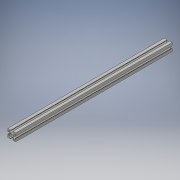
# Autodesk Inventor part: 20 in 80-20 extrusion
Saved by Autodesk Inventor 2016 SP2 (Build 200236200, 236)
## iProperties
Created: 2018-01-11
Part Number: 20 in 80-20 extrusion
Material: Generic
Document SubType Name: Modeling
Designer: CAD
Density: 1 g/cm^3
Appearance: Default
Author: CAD
Autodesk Inventor part; units mm, degrees
ref_plane "YZ Plane" through (0, 0, 0) normal (1, 0, 0) x (0, 1, 0)
ref_plane "XZ Plane" through (0, 0, 0) normal (0, 1, 0) x (-1, 0, 0)
ref_plane "XY Plane" through (0, 0, 0) normal (0, 0, 1) x (1, 0, 0)
sketch "Sketch1" plane through (0, 0, 0) normal (0, 0, 1) x (1, 0, 0)
  line L0 (-12.7, 12.7) -> (12.7, 12.7)
  line L1 (12.7, 12.7) -> (12.7, -12.7)
  line L2 (12.7, -12.7) -> (-12.7, -12.7)
  line L3 (-12.7, -12.7) -> (-12.7, 12.7)
  point P0 (0, 0)
  dimension "d0" = 25.4
  dimension "d1" = 25.4
  dimension "d2" = 12.7
  dimension "d3" = 12.7
  constraints: 8 end point, 2 parallel, 1 horizontal, 1 perpendicular
  measures "d0" distance of L1.end L2.end
  measures "d1" distance of L0.end L1.end
  measures "d2" distance from line of L1 point (0, 0)
  measures "d3" distance from line of point (0, 0) L0
extrude "Extrusion1" add sketch "Sketch1" along normal blind 508
sketch "Sketch2" plane through (0, 0, 508) normal (0, 0, 1) x (1, 0, 0)
  circle A0 centre (0, 0) radius 2.54
  line L0 (-4.5085, 4.5085) -> (4.5085, 4.5085)
  line L1 (-4.5085, -4.5085) -> (4.5085, -4.5085)
  line L2 (4.5085, 4.5085) -> (4.5085, -4.5085)
  line L3 (-4.5085, 4.5085) -> (-4.5085, -4.5085)
  line L4 (-3.0896, 4.5085) -> (-11.2811, 12.7)
  line L5 (-4.5085, 3.0537) -> (-12.7, 11.2452)
  line L6 (12.7, 12.7) -> (-12.7, 12.7) projected
  line L7 (-12.7, 12.7) -> (-12.7, 4.0005)
  line L8 (-10.668, 4.0005) -> (-10.668, 9.2132)
  line L9 (-9.2491, 10.668) -> (-3.3655, 10.668)
  line L10 (-12.7, 12.7) -> (-3.3655, 12.7)
  line L11 (-2.7305, 11.303) -> (-2.7305, 12.065)
  line L12 (-12.065, 3.3655) -> (-11.303, 3.3655)
  arc A1 (-12.7, 4.0005) -> (-12.065, 3.3655) centre (-12.065, 4.0005) ccw
  arc A2 (-11.303, 3.3655) -> (-10.668, 4.0005) centre (-11.303, 4.0005) ccw
  arc A3 (-3.3655, 10.668) -> (-2.7305, 11.303) centre (-3.3655, 11.303) ccw
  arc A4 (-2.7305, 12.065) -> (-3.3655, 12.7) centre (-3.3655, 12.065) ccw
  arc A5 (-3.3655, -11.303) -> (-4.0005, -10.668) centre (-4.0005, -11.303) ccw
  line L13 (-3.3655, -12.065) -> (-3.3655, -11.303)
  arc A6 (-4.0005, -12.7) -> (-3.3655, -12.065) centre (-4.0005, -12.065) ccw
  line L14 (-3.0537, -4.5085) -> (-11.2452, -12.7)
  line L15 (-10.668, -9.2491) -> (-10.668, -3.3655)
  line L16 (-4.5085, -3.0896) -> (-12.7, -11.2811)
  line L17 (-12.7, -12.7) -> (-12.7, -3.3655)
  arc A7 (-10.668, -3.3655) -> (-11.303, -2.7305) centre (-11.303, -3.3655) ccw
  line L18 (-11.303, -2.7305) -> (-12.065, -2.7305)
  arc A8 (-12.065, -2.7305) -> (-12.7, -3.3655) centre (-12.065, -3.3655) ccw
  line L19 (-4.0005, -10.668) -> (-9.2132, -10.668)
  line L20 (-12.7, -12.7) -> (-4.0005, -12.7)
  arc A9 (11.303, -3.3655) -> (10.668, -4.0005) centre (11.303, -4.0005) ccw
  line L21 (12.065, -3.3655) -> (11.303, -3.3655)
  arc A10 (12.7, -4.0005) -> (12.065, -3.3655) centre (12.065, -4.0005) ccw
  line L22 (4.5085, -3.0537) -> (12.7, -11.2452)
  line L23 (9.2491, -10.668) -> (3.3655, -10.668)
  line L24 (3.0896, -4.5085) -> (11.2811, -12.7)
  line L25 (12.7, -12.7) -> (3.3655, -12.7)
  arc A11 (3.3655, -10.668) -> (2.7305, -11.303) centre (3.3655, -11.303) ccw
  line L26 (2.7305, -11.303) -> (2.7305, -12.065)
  arc A12 (2.7305, -12.065) -> (3.3655, -12.7) centre (3.3655, -12.065) ccw
  line L27 (10.668, -4.0005) -> (10.668, -9.2132)
  line L28 (12.7, -12.7) -> (12.7, -4.0005)
  arc A13 (3.3655, 11.303) -> (4.0005, 10.668) centre (4.0005, 11.303) ccw
  line L29 (3.3655, 12.065) -> (3.3655, 11.303)
  arc A14 (4.0005, 12.7) -> (3.3655, 12.065) centre (4.0005, 12.065) ccw
  line L30 (3.0537, 4.5085) -> (11.2452, 12.7)
  line L31 (10.668, 9.2491) -> (10.668, 3.3655)
  line L32 (4.5085, 3.0896) -> (12.7, 11.2811)
  line L33 (12.7, 12.7) -> (12.7, 3.3655)
  arc A15 (10.668, 3.3655) -> (11.303, 2.7305) centre (11.303, 3.3655) ccw
  line L34 (11.303, 2.7305) -> (12.065, 2.7305)
  arc A16 (12.065, 2.7305) -> (12.7, 3.3655) centre (12.065, 3.3655) ccw
  line L35 (4.0005, 10.668) -> (9.2132, 10.668)
  line L36 (12.7, 12.7) -> (4.0005, 12.7)
  line L37 (-4.5085, 3.0537) -> (-4.5085, 4.5085)
  line L38 (-3.0896, 4.5085) -> (-4.5085, 4.5085)
  line L39 (-12.7, -12.7) -> (-4.0005, -12.7)
  line L40 (-4.0005, -10.668) -> (-9.2132, -10.668)
  line L41 (-10.668, -9.2491) -> (-10.668, -3.3655)
  line L42 (-12.7, -12.7) -> (-12.7, -3.3655)
  line L43 (-11.303, -2.7305) -> (-12.065, -2.7305)
  arc A17 (-10.668, -3.3655) -> (-11.303, -2.7305) centre (-11.303, -3.3655) ccw
  arc A18 (-12.065, -2.7305) -> (-12.7, -3.3655) centre (-12.065, -3.3655) ccw
  line L44 (-4.5085, -3.0896) -> (-4.5085, -4.5085)
  line L45 (-4.5085, -3.0896) -> (-12.7, -11.2811)
  line L46 (-3.0537, -4.5085) -> (-4.5085, -4.5085)
  line L47 (-3.0537, -4.5085) -> (-11.2452, -12.7)
  line L48 (-4.5085, -4.5085) -> (-4.5085, 4.5085)
  circle A19 centre (0, 0) radius 2.54
  line L49 (-4.5085, -4.5085) -> (4.5085, -4.5085)
  line L50 (-3.3655, -12.065) -> (-3.3655, -11.303)
  arc A20 (-4.0005, -12.7) -> (-3.3655, -12.065) centre (-4.0005, -12.065) ccw
  arc A21 (-3.3655, -11.303) -> (-4.0005, -10.668) centre (-4.0005, -11.303) ccw
  line L51 (12.7, -12.7) -> (12.7, -4.0005)
  line L52 (10.668, -4.0005) -> (10.668, -9.2132)
  line L53 (9.2491, -10.668) -> (3.3655, -10.668)
  line L54 (12.7, -12.7) -> (3.3655, -12.7)
  line L55 (2.7305, -11.303) -> (2.7305, -12.065)
  arc A22 (3.3655, -10.668) -> (2.7305, -11.303) centre (3.3655, -11.303) ccw
  arc A23 (2.7305, -12.065) -> (3.3655, -12.7) centre (3.3655, -12.065) ccw
  line L56 (3.0896, -4.5085) -> (4.5085, -4.5085)
  line L57 (3.0896, -4.5085) -> (11.2811, -12.7)
  line L58 (4.5085, -3.0537) -> (4.5085, -4.5085)
  line L59 (4.5085, -3.0537) -> (12.7, -11.2452)
  line L60 (4.5085, -4.5085) -> (-4.5085, -4.5085)
  circle A24 centre (0, 0) radius 2.54
  line L61 (4.5085, -4.5085) -> (4.5085, 4.5085)
  line L62 (12.065, -3.3655) -> (11.303, -3.3655)
  arc A25 (12.7, -4.0005) -> (12.065, -3.3655) centre (12.065, -4.0005) ccw
  arc A26 (11.303, -3.3655) -> (10.668, -4.0005) centre (11.303, -4.0005) ccw
  line L63 (12.7, 12.7) -> (4.0005, 12.7)
  line L64 (4.0005, 10.668) -> (9.2132, 10.668)
  line L65 (10.668, 9.2491) -> (10.668, 3.3655)
  line L66 (12.7, 12.7) -> (12.7, 3.3655)
  line L67 (11.303, 2.7305) -> (12.065, 2.7305)
  arc A27 (10.668, 3.3655) -> (11.303, 2.7305) centre (11.303, 3.3655) ccw
  arc A28 (12.065, 2.7305) -> (12.7, 3.3655) centre (12.065, 3.3655) ccw
  line L68 (4.5085, 3.0896) -> (4.5085, 4.5085)
  line L69 (4.5085, 3.0896) -> (12.7, 11.2811)
  line L70 (3.0537, 4.5085) -> (4.5085, 4.5085)
  line L71 (3.0537, 4.5085) -> (11.2452, 12.7)
  line L72 (4.5085, 4.5085) -> (4.5085, -4.5085)
  circle A29 centre (0, 0) radius 2.54
  line L73 (4.5085, 4.5085) -> (-4.5085, 4.5085)
  line L74 (3.3655, 12.065) -> (3.3655, 11.303)
  arc A30 (4.0005, 12.7) -> (3.3655, 12.065) centre (4.0005, 12.065) ccw
  arc A31 (3.3655, 11.303) -> (4.0005, 10.668) centre (4.0005, 11.303) ccw
  point P0 (-12.7, 3.3655)
  point P1 (-2.7305, 12.7)
  point P2 (-3.3655, -12.7)
  point P3 (-12.7, -2.7305)
  point P4 (12.7, -3.3655)
  point P5 (2.7305, -12.7)
  point P6 (3.3655, 12.7)
  point P7 (12.7, 2.7305)
  point P8 (-3.3655, -12.7)
  point P9 (-12.7, -2.7305)
  point P10 (12.7, -3.3655)
  point P11 (2.7305, -12.7)
  point P12 (3.3655, 12.7)
  point P13 (12.7, 2.7305)
  dimension "d6" = 5.08
  dimension "d7" = 9.017
  dimension "d8" = 4.5085
  dimension "d9" = 4.5085
  dimension "d10" = 4.5085
  dimension "d11" = 2.032
  dimension "d12" = 1.0033
  dimension "d13" = 135
  dimension "d17" = 9.3345
  dimension "d19" = 2.032
  dimension "d20" = 2.032
  dimension "d21" = 0.635
  dimension "d22" = 9.3345
  dimension "d25" = 360
  dimension "d29" = 360
  constraints: 148 end point, 59 point on line, 56 point on circle, 32 centre point, 8 tangent, 4 horizontal, 4 vertical, 3 coincident, 3 equal radius, 1 collinear, 1 parallel, 1 perpendicular, 300 other
  measures "d6" diameter of A0
  measures "d7" distance between parallel lines of L0 L1
  measures "d8" distance from line of L0 point (0, 0)
  measures "d9" distance from line of point (0, 0) L2
  measures "d10" distance from line of point (0, 0) L3
  measures "d11" distance between parallel lines of L5 L4
  measures "d12" distance from line of L0.start L4
  measures "d13" angle of L0 L4
  measures "d17" distance of L6.end point (-12.7, 3.365)
  measures "d19" distance between parallel lines of L7 L8
  measures "d20" distance between parallel lines of L6 L9
  measures "d21" radius of A1
  measures "d22" distance of L6.end L10.end
extrude "Extrusion2" cut sketch "Sketch2" against normal blind 1219.2 contours L3 L5 L7 L6 L4 L0 | L0 L2 L1 L3 | L30 L6 L33 L32 L2 L0 | L4 L6 A4 L11 A3 L9 | L3 L1 L14 L20 L17 L16 | L8 A2 L12 A1 L7 L5 | L35 A13 L29 A14 L6 L30 | L16 L17 A8 L18 A7 L15 | L22 L28 L25 L24 L1 L2 | L32 L33 A16 L34 A15 L31 | L19 A5 L13 A6 L20 L14 | L27 A9 L21 A10 L28 L22 | L24 L25 A12 L26 A11 L23 keep common part
equation "\"d22\" = d17"
body "Solid1"
